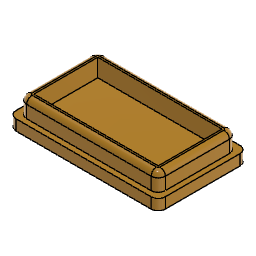
Alu-Leiter-Schuh-42x25_Einlage v3 (Autodesk Fusion 360 design; units mm, degrees)
Autodesk Fusion 360 part; units mm, degrees
sketch "Skizze1" plane through (0, 0, 0) normal (0, 0, 1) x (1, 0, 0)
  line L0 (0, 0) -> (42, 0)
  line L1 (42, 0) -> (42, 25)
  line L2 (42, 25) -> (0, 25)
  line L3 (0, 25) -> (0, 0)
  dimension "d1" = 42
  dimension "d2" = 25
  constraint horizontal L0
  constraint vertical L1
  constraint horizontal L2
  constraint vertical L3
  constraint coincident L0.start L3.end
  measures "d1" distance of L0.start L0.end
  measures "d2" distance of L0.start L2.end
extrude "Extrusion1" add sketch "Skizze1" along normal blind 3
sketch "Skizze2" plane through (0, 0, 3) normal (0, 0, 1) x (-1, 0, 0)
  line L0 (0, -25) -> (0, 0)
  line L1 (0, 0) -> (-42, 0)
  line L2 (-42, 0) -> (-42, -25)
  line L3 (-42, -25) -> (0, -25)
  line L4 (-40.5, -1.5) -> (-40.5, -23.5)
  line L5 (-40.5, -23.5) -> (-1.5, -23.5)
  line L6 (-1.5, -23.5) -> (-1.5, -1.5)
  line L7 (-1.5, -1.5) -> (-40.5, -1.5)
  line L8 (-38.4799, -3.5201) -> (-38.4799, -21.4799)
  line L9 (-38.4799, -21.4799) -> (-3.5201, -21.4799)
  line L10 (-3.5201, -21.4799) -> (-3.5201, -3.5201)
  line L11 (-3.5201, -3.5201) -> (-38.4799, -3.5201)
  dimension "d6" = -1.5
  dimension "d7" = -3.5201
extrude "Extrusion2" add sketch "Skizze2" along normal blind 5 contours L4 L5 L6 L7
fillet "Abrundung1" radius 2 8 edges at (0, 25, 1.5) (1.5, 23.5, 5.5) (40.5, 23.5, 5.5) (42, 25, 1.5) (0, 0, 1.5) (1.5, 1.5, 5.5) (40.5, 1.5, 5.5) (42, 0, 1.5)
fillet "Abrundung2" radius 1.5 8 edges at (39.9142, 2.0858, 8) (40.5, 12.5, 8) (39.9142, 22.9142, 8) (21, 23.5, 8) (2.0858, 22.9142, 8) (1.5, 12.5, 8) (2.0858, 2.0858, 8) (21, 1.5, 8)
